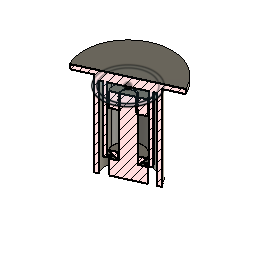
TireLabelStick_V2 (Autodesk Fusion 360 design; units mm, degrees)
part number: 2025-11-17-07-45-38-028
Autodesk Fusion 360 part; units mm, degrees
sketch "StickSketch" plane through (0, 0, 0) normal (0, 0, 1) x (1, 0, 0)
  circle A0 centre (0, 0) radius 5
  circle A1 centre (0, 0) radius 10
  dimension "d1" = 10
  dimension "d4" = 20
  constraint coincident A0.centre A1.centre
  measures "d1" diameter of A0
  measures "d4" diameter of A1
extrude "Extrude1" add sketch "StickSketch" along normal blind 50 contours A0 makes body 1
extrude "Extrude2" add sketch "StickSketch" along normal blind 10 bodies 1
sketch "StickTopSketch" plane through (0, 0, 50) normal (0, 0, 1) x (-1, 0, 0)
  circle A0 centre (0, 0) radius 5
  circle A1 centre (0, 0) radius 10
  dimension "d7" = 20
  constraint concentric A0 A1
  measures "d7" diameter of A1
extrude "Extrude3" add sketch "StickTopSketch" against normal blind 10 separate body makes body 2
sketch "MovingPart" plane through (0, 0, 10) normal (0, 0, 1) x (-1, 0, 0)
  circle A0 centre (0, 0) radius 5
  circle A1 centre (0, 0) radius 10
  circle A2 centre (0, 0) radius 5.2
  circle A3 centre (0, 0) radius 10
  dimension "d17" = 10.4
  dimension "d18" = 20
  constraint concentric A0 A2
  constraint concentric A0 A3
  measures "d17" diameter of A2
  measures "d18" diameter of A3
extrude "Extrude4" add sketch "MovingPart" along normal blind 5 separate body contours A1 A3 makes body 3
chamfer "Chamfer1" distance 4.8 angle 45 1 edges at (9.3233, 3.6162, 10) on bodies 3
ref_plane "WorkPlane1" through (0, 0, 30) normal (0, 1, 0) x (0, 0, 1)
sketch "LockSketch" plane through (0, 0, 0) normal (0, 1, 0) x (1, 0, 0)
  line L0 (-13, -55) -> (-11, -55)
  line L1 (-11, -55) -> (-11, -10.5)
  line L2 (-11, -10.5) -> (-13, -10.5)
  line L3 (-13, -10.5) -> (-13, -55)
  line L4 (-11, -12) -> (-7.5, -12)
  line L5 (-7.5, -12) -> (-11, -10.5)
  line L6 (0, 10) -> (0, -70)
  line L7 (13, -55) -> (11, -55)
  line L8 (11, -12) -> (7.5, -12)
  line L9 (11, -10.5) -> (13, -10.5)
  line L10 (13, -10.5) -> (13, -55)
  line L11 (11, -55) -> (11, -10.5)
  line L12 (7.5, -12) -> (11, -10.5)
  dimension "d23" = 44.5
  dimension "d24" = 3.5
  constraint horizontal L0
  constraint vertical L1
  constraint horizontal L2
  constraint vertical L3
  constraint coincident L1 L4.start
  constraint perpendicular L1 L4
  constraint symmetric L0.start L6 L7.start
  constraint symmetric L0.end L6 L7.end
  constraint symmetric L1.end L6 L9.start
  constraint symmetric L2.end L6 L9.end
  constraint symmetric L4.start L6 L8.start
  constraint symmetric L4.end L6 L8.end
  measures "d23" distance of L0.start L2.end
  measures "d24" distance of L4.start L4.end
revolve "Revolve1" add sketch "LockSketch" angle 40 about axis through (0, 0, -10) along (0, 0, 1) separate body makes body 4 at (12.1092, 4.7293, 25.3333) makes body 5 at (-12.1092, -4.7293, 25.3333)
sketch "CoverSketch" plane through (0, 0, 55) normal (0, 0, 1) x (-1, 0, 0)
  line L0 (11, 0) -> (13, 0)
  arc A0 (13, 0) -> (9.9586, 8.3562) centre (0, 0) ccw
  line L1 (9.9586, 8.3562) -> (8.4265, 7.0707)
  arc A1 (11, 0) -> (8.4265, 7.0707) centre (0, 0) ccw
  circle A2 centre (0, 0) radius 17.5
  circle A3 centre (0, 0) radius 15
  dimension "d27" = 35
  dimension "d28" = 30
  constraint concentric A0 A2
  constraint concentric A2 A3
  measures "d27" diameter of A2
  measures "d28" diameter of A3
extrude "Extrude5" add sketch "CoverSketch" along normal blind 3 contours L0 A0 L1 A1 | A2 | A3 bodies 4 5
extrude "Extrude6" add sketch "CoverSketch" against normal blind 55 contours A2 bodies 4
move_face "OffsetFaces6" offset -0.1 1 faces at (4.9752, -0.4978, 23.3333) on bodies 1
thread "Thread7" "ISO Metric profile 10.0 M10x1.5 M10x1.5 6H" major diameter 10.198 minor diameter 8.526 pitch 1.5 angle 60 modelled right hand crest width 0.4094 on face at (-4.9938, 0.2492, 43.3333) from (0, 0, 50) to (0, 0, 40) crest through (-4.263, 0, 49.625) on bodies 2
thread "Thread8" "ISO Metric profile 10.0 M10x1.5 M10x1.5 6g" major diameter 9.85 minor diameter 8.141 pitch 1.5 angle 60 modelled right hand crest width 0.2177 on face at (4.8939, 0.2442, 23.3333) from (0, 0, 40) to (0, 0, 50) crest through (4.925, 0, 9.625) on bodies 1
sketch "Sketch7" plane through (0, 0, 58) normal (0, 0, 1) x (-1, 0, 0)
  circle A0 centre (0, 0) radius 17.5
  circle A1 centre (0, 0) radius 30
  dimension "d48" = 60
  constraint concentric A0 A1
  measures "d48" diameter of A1
extrude "Extrude7" add sketch "Sketch7" along normal blind 3 contours A0 | A1 bodies 4
named bodies: "Stick", "StickTop", "MovingPart", "Cover"
